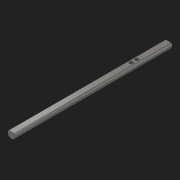
# Autodesk Inventor part: 6mm x 160mm D Shaft
Saved by Autodesk Inventor 2017 SP1 (Build 210196100, 196)
## iProperties
Created: 2018-04-13
Part Number: 6mm x 160mm D Shaft
Material: Stainless Steel
Document SubType Name: Modeling
Designer: Zach
Density: 8 g/cm^3
Appearance: Semi-Polished
Author: Zach
Autodesk Inventor part; units mm, degrees
ref_plane "YZ Plane" through (0, 0, 0) normal (1, 0, 0) x (0, 1, 0)
ref_plane "XZ Plane" through (0, 0, 0) normal (0, 1, 0) x (-1, 0, 0)
ref_plane "XY Plane" through (0, 0, 0) normal (0, 0, 1) x (1, 0, 0)
sketch "Sketch1" plane through (0, 0, 0) normal (0, 0, 1) x (1, 0, 0)
  circle A0 centre (0, 0) radius 3 construction
  line L0 (-2.2361, 2) -> (2.2361, 2)
  arc A1 (-2.2361, 2) -> (2.2361, 2) centre (0, 0) ccw
  dimension "d0" = 6
  dimension "d1" = 2
  constraints: 4 point on circle, 2 centre point, 2 end point, 1 coincident, 1 concentric, 1 horizontal
  measures "d0" diameter of A0
  measures "d1" distance from line of L0 point (0, 0)
extrude "Extrusion1" add sketch "Sketch1" along normal blind 130
sketch "Sketch2" plane through (-2.2361, 2, 0) normal (0, 1, 0) x (1, 0, 0)
  circle A0 centre (2.2361, -127.9) radius 1.45
  line L0 (4.4721, -130) -> (0, -130) projected
  circle A1 centre (2.2361, -26.2) radius 1.45
  line L1 (0, 0) -> (4.4721, 0) projected
  circle A2 centre (2.2361, -30.8) radius 1.45
  circle A3 centre (2.2361, -123.3) radius 1.45
  point P0 (2.2361, 0)
  point P1 (2.2361, -130)
  point P2 (2.2361, 0)
  dimension "d4" = 2.9
  dimension "d5" = 2.1
  dimension "d8" = 2.9
  dimension "d9" = 26.2
  dimension "d10" = 2.9
  dimension "d11" = 4.6
  dimension "d12" = 2.9
  dimension "d13" = 4.6
  constraints: 4 centre point, 4 vertical alignment, 2 midpoint
  measures "d4" diameter of A0
  measures "d5" distance from line of L0 A0.centre
  measures "d8" diameter of A1
  measures "d9" distance from line of A1.centre L1
  measures "d10" diameter of A2
  measures "d11" distance of A2.centre A1.centre
  measures "d12" diameter of A3
  measures "d13" distance of A0.centre A3.centre
extrude "Extrusion2" cut sketch "Sketch2" against normal through all contours A1 | A2
thread "Thread3" size "M3x0.5" class "6H" standard "ANSI Metric M Profile" full length
thread "Thread4" size "M3x0.5" class "6H" standard "ANSI Metric M Profile" full length
body "Solid1"
